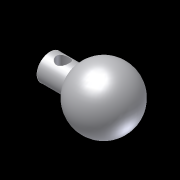
# Autodesk Inventor part: Glocke02
Saved by Autodesk Inventor 2013 (Build 170138000, 138)
## iProperties
Created: 2005-03-10
Part Number: Glocke02
Document SubType Name: Modeling
Designer: acad
Manufacturer: Standard
Standards Organization: Custom
Material: Allgemein
Density: 1 g/cm^3
Author: acad
Autodesk Inventor part; units mm, degrees
ref_plane "YZ Plane" through (0, 0, 0) normal (1, 0, 0) x (0, 1, 0)
ref_plane "XZ Plane" through (0, 0, 0) normal (0, 1, 0) x (-1, 0, 0)
ref_plane "XY Plane" through (0, 0, 0) normal (0, 0, 1) x (1, 0, 0)
sketch "Skizze1" plane through (0, 0, 0) normal (0, 0, 1) x (1, 0, 0)
  line L0 (1.6815, 1.335) -> (21.0061, 1.335)
  arc A0 (21.0061, 1.335) -> (7.6815, 4.335) centre (14.0061, 1.335) ccw
  line L1 (1.6815, 4.335) -> (1.6815, 1.335)
  line L2 (1.6815, 4.335) -> (7.6815, 4.335)
  dimension "d2" = 6
  dimension "d4" = 7
  dimension "d14" = 6
  constraints: 6 end point, 2 perpendicular, 2 point on circle, 1 centre point, 1 horizontal, 1 point on line
  measures "d2" diameter of L2 L0
  measures "d4" radius of A0
  measures "d14" distance of L1.start L2.end
revolve "Drehung1" add sketch "Skizze1" angle 360 about axis through (1.6815, 1.335, 0) along (1, 0, 0)
ref_plane "Arbeitsebene1" through (4.6815, 1.335, -3) normal (0, 0, 1) x (1, 0, 0)
sketch "Skizze2" plane through (4.6815, 1.335, -3) normal (0, 0, 1) x (1, 0, 0)
  line L0 (-3, -3) -> (-3, 3) projected
  line L1 (-3, -3) -> (3, -3) projected
  point P0 (0, 0)
  dimension "d5" = 3
  dimension "d6" = 3
  measures "d5" distance from line of L0 point (0, 0)
  measures "d6" distance from line of point (0, 0) L1
hole "Bohrung1" at (4.6815, 1.335, -3) direction (0, 0, 1) diameter 3 end through all
